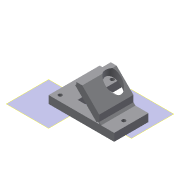
# Autodesk Inventor part: cellSTORM_dichroic_mirror_adjuster_tmp
Saved by Autodesk Inventor 2019.4 (Build 234330000, 330)
## iProperties
Created: 2020-06-30
Part Number: cellSTORM_dichroic_mirror_adjuster_tmp
Material: Generic
Document SubType Name: Modeling
Designer: diederichbenedict
Density: 1 g/cm^3
Appearance: Default
Author: diederichbenedict
Autodesk Inventor part; units mm, degrees
ref_plane "YZ Plane" through (0, 0, 0) normal (1, 0, 0) x (0, 1, 0)
ref_plane "XZ Plane" through (0, 0, 0) normal (0, 1, 0) x (-1, 0, 0)
ref_plane "XY Plane" through (0, 0, 0) normal (0, 0, 1) x (1, 0, 0)
ref_plane "Work Plane12" through (-3.3573, 3.9, 0.05) normal (0, -1, 0) x (1, 0, 0)
sketch "Sketch16" plane through (-3.3573, 3.9, 0.05) normal (0, -1, 0) x (1, 0, 0)
  circle A0 centre (-22.9842, 13.95) radius 1
  circle A1 centre (-16.4842, -6.55) radius 1
  circle A2 centre (5.0158, 8.95) radius 1
  line L0 (-25.9842, 16.95) -> (8.0158, 16.95)
  line L1 (8.0158, 16.95) -> (8.0158, -0.8439)
  line L2 (8.0158, -0.8439) -> (-14.4842, -0.8439)
  line L3 (-25.9842, -0.8439) -> (-25.9842, 16.95)
  line L4 (-14.4842, -0.8439) -> (-14.4842, -9.55)
  line L5 (-14.4842, -9.55) -> (-25.9842, -9.55)
  line L6 (-25.9842, -9.55) -> (-25.9842, -0.8439)
  circle A3 centre (-5.4842, 3.95) radius 2.6486 construction
  line L7 (-16.2963, 11.5695) -> (-1.2963, 11.5695)
  line L8 (-1.2963, 11.5695) -> (-1.2963, 0.5695)
  line L9 (-1.2963, 0.5695) -> (-16.2963, 0.5695)
  line L10 (-16.2963, 0.5695) -> (-16.2963, 11.5695)
  line L11 (-16.2963, 11.5695) -> (-1.2963, 0.5695) construction
  line L12 (-1.2963, 11.5695) -> (-16.2963, 0.5695) construction
  point P0 (5.0158, 8.95)
  point P1 (-22.9842, 13.95)
  point P2 (-8.7963, 6.0695)
  point P3 (-14.4842, -0.8439)
  point P4 (-14.4842, -0.8439)
  dimension "d73" = 3
  dimension "d74" = 3
  dimension "d75" = 3
  dimension "d76" = 2
  dimension "d77" = 3
  dimension "d80" = 15
  dimension "d81" = 11
  constraints: 26 end point, 5 parallel, 4 centre point, 3 coincident, 2 horizontal, 2 midpoint, 2 perpendicular, 8 other
  measures "d73" distance from line of A0.centre L0
  measures "d74" distance from line of A0.centre L3
  measures "d75" distance from line of L5 A1.centre
  measures "d76" distance from line of L4 A1.centre
  measures "d77" distance from line of L1 point (5.016, 8.95)
  measures "d80" distance of L8.end L9.end
  measures "d81" distance of L7.end L8.end
extrude "Extrusion15" add sketch "Sketch16" against normal blind 4
ref_plane "Work Plane6" through (-29.3415, 3.9, 17) normal (0, -1, 0) x (1, 0, 0)
sketch "Sketch22" plane through (4.6585, 3.9, -0.7939) normal (0, 0, -1) x (-1, 0, 0)
  line L0 (18.839, 15.3533) -> (7.5253, 4.0395) construction
  line L1 (8.2324, 3.3324) -> (19.5461, 14.6461) construction
  line L2 (7.5253, 4.0395) -> (19.5461, 16.0604)
  line L3 (19.5461, 16.0604) -> (19.5461, 17.0604)
  line L4 (34, 4) -> (0, 4) projected
  line L5 (19.5461, 17.0604) -> (16.5461, 17.0604)
  line L6 (16.5461, 17.0604) -> (7.7787, 8.2929)
  line L7 (7.7787, 8.2929) -> (7.7787, 5)
  line L8 (7.7787, 5) -> (6.7787, 4)
  line L9 (7.5253, 4.0395) -> (7.4858, 4)
  line L10 (7.4858, 4) -> (6.7787, 4)
  line L11 (18.839, 15.3533) -> (19.5461, 14.6461)
  point P0 (4.6585, -3.9)
  dimension "d82" = 135
  dimension "d83" = 3
  dimension "d84" = 1
  dimension "d85" = 1
  dimension "d86" = 1
  dimension "d87" = 0.5
  constraints: 22 end point, 3 point on line, 2 parallel, 2 perpendicular, 7 other
  measures "d82" angle of L8 L7
  measures "d83" distance of L3.end L5.end
  measures "d84" distance of L2.end L3.end
  measures "d85" horizontal distance of L8.end L7.end
  measures "d86" distance from line of L11 L2.end
  measures "d87" distance between parallel lines of L8 L0
ref_plane "Work Plane18" through (17.1585, 14, 21) normal (0, 0, 1) x (1, 0, 0)
extrude "Extrusion21" add sketch "Sketch22" against normal up to surface (17.7939 mm away)
sketch "Sketch23" plane through (-3.3573, 3.9, 0.05) normal (0, -1, 0) x (1, 0, 0)
  circle A0 centre (-5.4842, 3.95) radius 2
  circle A1 centre (-5.4842, 3.95) radius 4
  point P0 (3.3573, -0.05)
  dimension "d90" = 8
  constraints: 2 centre point, 1 coincident, 2 other
  measures "d90" diameter of A1
extrude "Extrusion22" cut sketch "Sketch23" against normal through all contours A0 | A1
sketch "Sketch24" plane through (-14.8876, 19.9604, 17) normal (-0.7071068, -0.7071068, 0) x (-0.7071068, 0.7071068, 0)
  circle A0 centre (-9, 13) radius 8 construction
  circle A1 centre (-7.713, 13) radius 8.1
  line L0 (0, 17.7939) -> (0, 0) construction
  line L1 (-17.0559, 17.7939) -> (0, 17.7939) construction
  line L2 (-1.184, 17.7939) -> (0, 17.7939) construction
  line L3 (0, 15.4738) -> (0, 17.7939)
  line L4 (0, 17.7939) -> (-1.184, 17.7939)
  line L5 (-14.242, 17.7939) -> (-15.813, 17.7939)
  line L6 (0, 10.5262) -> (0, 0)
  line L7 (-8.5505, 9) -> (-5.7221, 9) projected
  line L8 (-17.0559, 0) -> (0, 0) projected
  line L9 (-17.0559, 0) -> (-17.0559, 17.7939) projected
  line L10 (0, 0) -> (-15.813, 0)
  line L11 (-13.8133, 17.7939) -> (-16.1417, 17.7939) projected
  line L12 (-15.813, 17.7939) -> (-15.813, -0.0523)
  point P0 (-24.6412, 17)
  dimension "d93" = 16.2
  constraints: 14 end point, 6 point on line, 4 point on circle, 3 collinear, 3 perpendicular, 2 centre point, 1 horizontal, 1 tangent, 2 other
  measures "d93" diameter of A1
extrude "Extrusion23" add sketch "Sketch24" along normal blind 1 contours A1 L4 L3 | L6 L8 L12 A1 | L12 L5 A1
sketch "Sketch25" plane through (4.6585, 3.9, -0.7939) normal (0, 0, -1) x (-1, 0, 0)
  line L0 (0, 0) -> (22.5, 0) projected
  line L1 (22.5, 0) -> (22.5, 4) projected
  line L2 (7.4858, 4) -> (22.5, 4) projected
  line L3 (7.4858, 4) -> (8.3647, 4.8789) projected
  line L4 (8.3647, 4.8789) -> (9.0718, 4.1718) projected
  line L5 (10.1826, 5.2826) -> (9.0718, 4.1718) projected
  line L6 (9.4755, 5.9897) -> (10.1826, 5.2826) projected
  line L7 (9.4755, 5.9897) -> (18.7089, 15.2232) projected
  line L8 (18.7089, 15.2232) -> (19.4161, 14.5161) projected
  line L9 (20.2533, 15.3533) -> (19.4161, 14.5161) projected
  line L10 (19.5461, 16.0604) -> (20.2533, 15.3533) projected
  line L11 (19.5461, 16.0604) -> (19.5461, 17.0604) projected
  line L12 (19.5461, 17.0604) -> (16.5461, 17.0604) projected
  line L13 (16.5461, 17.0604) -> (7.7787, 8.2929) projected
  line L14 (7.7787, 8.2929) -> (7.7787, 5) projected
  line L15 (7.7787, 5) -> (6.7787, 4) projected
  line L16 (0, 4) -> (6.7787, 4) projected
  line L17 (0, 0) -> (0, 4) projected
  line L18 (8.3647, 4.8789) -> (9.4755, 5.9897) projected
  line L19 (8.3647, 4.8789) -> (10.1826, 5.2826)
  line L20 (10.1826, 5.2826) -> (9.0718, 4.1718) projected
  point P0 (4.6585, -3.9)
  constraints: 2 end point, 2 point on line
extrude "Extrusion24" cut sketch "Sketch25" against normal through all contours L19 L5 L4
sketch "Sketch26" plane through (-15.5947, 19.2533, 17) normal (-0.7071068, -0.7071068, 0) x (0, 0, -1)
  line L0 (8.2061, 14.242) -> (0, 14.242) projected
  line L1 (0, 14.242) -> (0, 0) projected
  line L2 (0, 0) -> (10.5262, 0) projected
  arc A0 (8.2061, 14.242) -> (10.5262, 0) centre (13, 7.713) ccw projected
  circle A1 centre (13, 7.713) radius 7.7907
  line L3 (8.2061, 14.242) -> (0, 14.242) projected
  line L4 (8.2061, 14.242) -> (8.7496, 14.242)
  line L5 (10.5262, 0) -> (11.9028, 0)
  point P0 (17, 24.6412)
  constraints: 4 end point, 3 point on circle, 2 point on line, 1 centre point, 1 coincident, 1 horizontal
extrude "Extrusion25" add sketch "Sketch26" along normal blind 0.5 contours A0 L2 L1 L0 | L4 A1 L5 A0
sketch "Sketch27" plane through (-19.6536, 3.9, 0.6195) normal (1, 0, 0) x (0, 0, -1)
  line L0 (0, 0) -> (-11, 0) projected
  line L1 (0, 0) -> (0, 4) projected
  line L2 (-11, 4) -> (0, 4) projected
  line L3 (-11, 0) -> (-11, 4) projected
  line L4 (-16.3805, 0) -> (-10.3805, 0)
  line L5 (-10.3805, 0) -> (-10.3805, 17)
  line L6 (-10.3805, 17) -> (-16.3805, 17)
  line L7 (-16.3805, 17) -> (-16.3805, 0)
  circle A0 centre (-13.7515, 14.9104) radius 1.45
  point P0 (0.6195, -3.9)
  point P1 (-16.3805, 0)
  dimension "d100" = 6
  dimension "d101" = 17
  dimension "d102" = 2.9
  constraints: 8 end point, 2 parallel, 1 centre point, 1 coincident, 1 horizontal, 1 perpendicular
  measures "d100" distance of L6.end L5.end
  measures "d101" distance of L5.end L4.end
  measures "d102" diameter of A0
extrude "Extrusion26" add sketch "Sketch27" against normal blind 3 contours L0 L3 L2 L5 | L4 L7 L6 L5 L2 L3
chamfer "Chamfer1" distance 2 angle 45 2 edges at (-19.6536, 7.9, 14.3097) (-22.6536, 7.9, 14)
sketch "Sketch28" plane through (-14.8876, 20.9604, -0.7939) normal (-1, 0, 0) x (0, 0, 1)
  circle A0 centre (15.1649, -2.15) radius 1.45 projected
  circle A1 centre (15.1649, -2.15) radius 1.95
  point P0 (0.7939, -20.9604)
  dimension "d108" = 0.5
  constraints: 1 centre point
  measures "d108" radial gap between concentric circles of A0 A1
extrude "Extrusion27" cut sketch "Sketch28" along normal blind 3 contours A0 | A1
body "Solid1"
